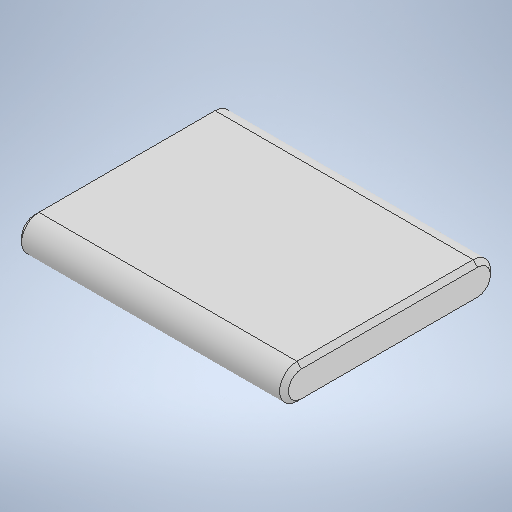
# Autodesk Inventor part: Domino2
Saved by Autodesk Inventor 2025.3 (Build 293356000, 356)
## iProperties
Created: 2025-11-20
Part Number: Domino2
Material: Generic
Document SubType Name: Modeling
Designer: User
Density: 1 g/cm^3
Appearance: Default
Author: User
Autodesk Inventor part; units mm, degrees
ref_plane "YZ Plane" through (0, 0, 0) normal (1, 0, 0) x (0, 1, 0)
ref_plane "XZ Plane" through (0, 0, 0) normal (0, 1, 0) x (-1, 0, 0)
ref_plane "XY Plane" through (0, 0, 0) normal (0, 0, 1) x (1, 0, 0)
sketch "Sketch1" plane through (0, 0, 0) normal (1, 0, 0) x (0, 1, 0)
  line L0 (0, 9.9) -> (0, -9.9) construction
  line L1 (-1.95, 9.9) -> (-1.95, -9.9)
  line L2 (1.95, -9.9) -> (1.95, 9.9)
  arc A0 (1.95, 9.9) -> (-1.95, 9.9) centre (0, 9.9) ccw
  arc A1 (-1.95, -9.9) -> (1.95, -9.9) centre (0, -9.9) ccw
  point P0 (0, 0)
  dimension "d0" = 9.9
  dimension "d1" = 3.9
  constraints: 8 end point, 4 point on circle, 4 tangent, 2 centre point, 1 midpoint, 1 parallel, 1 vertical
  measures "d0" distance of point (0, 0) L0.end
  measures "d1" diameter of A1
extrude "Extrusion1" add sketch "Sketch1" along normal mid plane 30
chamfer "Chamfer1" distance 0.5 angle 45 8 edges at (-15, 1.95, 0) (-15, 0, -11.85) (-15, -1.95, 0) (-15, 0, 11.85) (15, 1.95, 0) (15, 0, 11.85) (15, -1.95, 0) (15, 0, -11.85)
body "Solid1"
